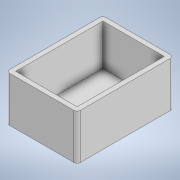
# Autodesk Inventor part: Case RevA
Saved by Autodesk Inventor 2021 (Build 250183000, 183)
## iProperties
Created: 2021-07-23
Part Number: Case RevA
Material: Generic
Document SubType Name: Modeling
Designer: cmzgt
Density: 1 g/cm^3
Appearance: Default
Author: cmzgt
Autodesk Inventor part; units mm, degrees
ref_plane "YZ Plane" through (0, 0, 0) normal (1, 0, 0) x (0, 1, 0)
ref_plane "XZ Plane" through (0, 0, 0) normal (0, 1, 0) x (-1, 0, 0)
ref_plane "XY Plane" through (0, 0, 0) normal (0, 0, 1) x (1, 0, 0)
sketch "Sketch1" plane through (0, 0, 0) normal (0, 1, 0) x (-1, 0, 0)
  line L0 (0, 0) -> (67, 0)
  line L1 (67, 0) -> (67, -91.44)
  line L2 (67, -91.44) -> (0, -91.44)
  line L3 (0, -91.44) -> (0, 0)
  dimension "d0" = 91.44
  dimension "d1" = 67
  constraints: 8 end point, 2 parallel, 1 horizontal, 1 perpendicular
  measures "d0" distance of L0.end L1.end
  measures "d1" distance of L1.end L2.end
extrude "Extrusion1" add sketch "Sketch1" along normal blind 3.81
sketch "Sketch3" plane through (0, 3.81, 0) normal (0, 1, 0) x (1, 0, 0)
  line L0 (-67, 0) -> (0, 0) projected
  line L1 (0, 91.44) -> (-67, 91.44) projected
  line L2 (-67, 0) -> (-59.535, 0)
  line L3 (-62.555, 4.445) -> (-62.555, 86.995)
  line L4 (-62.555, 91.44) -> (-67, 91.44)
  line L5 (-67, 91.44) -> (-67, 0)
  line L6 (-33.5, 0) -> (-33.5, 91.44) construction
  line L7 (-59.535, 0) -> (-33.5, 0)
  line L8 (-33.5, 4.445) -> (-62.555, 4.445)
  line L9 (-62.555, 91.44) -> (-33.5, 91.44)
  line L10 (-33.5, 86.995) -> (-62.555, 86.995)
  line L11 (0, 0) -> (-67, 0)
  line L12 (0, 0) -> (-7.465, 0)
  line L13 (-4.445, 4.445) -> (-4.445, 86.995)
  line L14 (-4.445, 91.44) -> (0, 91.44)
  line L15 (0, 91.44) -> (0, 0)
  line L16 (-33.5, 4.445) -> (-4.445, 4.445)
  line L17 (-4.445, 91.44) -> (-33.5, 91.44)
  line L18 (-33.5, 86.995) -> (-4.445, 86.995)
  dimension "d25" = 4.445
  dimension "d27" = 4.445
  dimension "d28" = 4.445
  dimension "d30" = 26.035
  dimension "d31" = 4.445
  dimension "d32" = 86.995
  dimension "d33" = 4.445
  constraints: 34 end point, 7 symmetric about line, 4 parallel, 3 horizontal, 3 point on line, 2 midpoint, 1 perpendicular
  measures "d25" distance of L8.start L7.end
  measures "d27" distance of L9.end L10.start
  measures "d28" distance between parallel lines of L5 L3
  measures "d30" distance of L6.start L2.end
  measures "d31" distance between parallel lines of L18 L1
  measures "d32" distance between parallel lines of L16 L1
  measures "d33" distance from line of L17.start L15
extrude "Extrusion2" add sketch "Sketch3" along normal blind 39
fillet "Fillet1" radius 3.175 4 edges at (-67, 21.405, -91.44) (-67, 21.405, 0) (0, 21.405, 0) (0, 21.405, -91.44)
body "Solid1"
